Autodesk Inventor part; units mm, degrees
(part 4 of 4)
  arc A561 (-1.6111, 29.8706) -> (-1.4437, 30.2273) centre (-7.325, 32.7708) ccw
  arc A562 (-1.4437, 30.2273) -> (-1.2651, 30.6794) centre (-8.4075, 33.2394) ccw
  arc A563 (-1.2651, 30.6794) -> (-1.5585, 30.9505) centre (-15.3265, 15.7621) ccw
  arc A564 (-1.5585, 30.9505) -> (-1.9952, 30.737) centre (1.554, 24.031) ccw
  arc A565 (-1.9952, 30.737) -> (-2.3376, 30.5421) centre (1.0019, 25.0734) ccw
  arc A566 (-2.3376, 30.5421) -> (-2.5999, 30.3711) centre (0.4096, 26.0425) ccw
  arc A567 (-2.5999, 30.3711) -> (-2.8883, 30.6174) centre (-15.3265, 15.7621) ccw
  arc A568 (-2.8883, 30.6174) -> (-2.7604, 30.9032) centre (-7.6343, 32.9126) ccw
  arc A569 (-2.7604, 30.9032) -> (-2.6214, 31.2719) centre (-8.6842, 33.3461) ccw
  arc A570 (-2.6214, 31.2719) -> (-2.4789, 31.7366) centre (-9.8001, 33.7284) ccw
  arc A571 (-2.4789, 31.7366) -> (-2.7926, 31.984) centre (-15.3265, 15.7621) ccw
  arc A572 (-2.7926, 31.984) -> (-3.2112, 31.7368) centre (0.8532, 25.33) ccw
  arc A573 (-3.2112, 31.7368) -> (-3.5372, 31.5157) centre (0.221, 26.3258) ccw
  arc A574 (-3.5372, 31.5157) -> (-3.7853, 31.3246) centre (-0.4455, 27.2455) ccw
  arc A575 (-3.7853, 31.3246) -> (-4.0922, 31.5475) centre (-15.3265, 15.7621) ccw
  arc A576 (-4.0922, 31.5475) -> (-3.9871, 31.8425) centre (-9.0037, 33.4633) ccw
  arc A577 (-3.9871, 31.8425) -> (-3.8775, 32.2209) centre (-10.0843, 33.8131) ccw
  arc A578 (-3.8775, 32.2209) -> (-3.7718, 32.6954) centre (-11.2268, 34.1066) ccw
  arc A579 (-3.7718, 32.6954) -> (-4.104, 32.9173) centre (-15.3265, 15.7621) ccw
  arc A580 (-4.104, 32.9173) -> (-4.5019, 32.6381) centre (0.0527, 26.5699) ccw
  arc A581 (-4.5019, 32.6381) -> (-4.8096, 32.3921) centre (-0.6557, 27.5131) ccw
  arc A582 (-4.8096, 32.3921) -> (-5.0419, 32.1821) centre (-1.3924, 28.3776) ccw
  arc A583 (-5.0419, 32.1821) -> (-5.3653, 32.3803) centre (-15.3265, 15.7621) ccw
  arc A584 (-5.3653, 32.3803) -> (-5.2837, 32.6826) centre (-10.412, 33.9048) ccw
  arc A585 (-5.2837, 32.6826) -> (-5.2041, 33.0685) centre (-11.5167, 34.1687) ccw
  arc A586 (-5.2041, 33.0685) -> (-5.136, 33.5498) centre (-12.6787, 34.3717) ccw
  arc A587 (-5.136, 33.5498) -> (-5.4845, 33.745) centre (-15.3265, 15.7621) ccw
  arc A588 (-5.4845, 33.745) -> (-5.8594, 33.4354) centre (-0.8427, 27.7432) ccw
  arc A589 (-5.8594, 33.4354) -> (-6.1468, 33.166) centre (-1.6229, 28.628) ccw
  arc A590 (-6.1468, 33.166) -> (-6.3619, 32.9384) centre (-2.4252, 29.432) ccw
  arc A591 (-6.3619, 32.9384) -> (-6.6999, 33.1106) centre (-15.3265, 15.7621) ccw
  arc A592 (-6.6999, 33.1106) -> (-6.6422, 33.4184) centre (-11.8506, 34.2345) ccw
  arc A593 (-6.6422, 33.4184) -> (-6.5932, 33.8093) centre (-12.9726, 34.4109) ccw
  arc A594 (-6.5932, 33.8093) -> (-6.563, 34.2945) centre (-14.147, 34.5221) ccw
  arc A595 (-6.563, 34.2945) -> (-6.9258, 34.4617) centre (-15.3265, 15.7621) ccw
  arc A596 (-6.9258, 34.4617) -> (-7.2752, 34.1237) centre (-1.8274, 28.8427) ccw
  arc A597 (-7.2752, 34.1237) -> (-7.5406, 33.8326) centre (-2.6746, 29.6635) ccw
  arc A598 (-7.5406, 33.8326) -> (-7.7372, 33.5888) centre (-3.5375, 30.4021) ccw
  arc A599 (-7.7372, 33.5888) -> (-8.0876, 33.7339) centre (-15.3265, 15.7621) ccw
  arc A600 (-8.0876, 33.7339) -> (-8.0543, 34.0453) centre (-13.3106, 34.4503) ccw
  arc A601 (-8.0543, 34.0453) -> (-8.0361, 34.4389) centre (-14.443, 34.5381) ccw
  arc A602 (-8.0361, 34.4389) -> (-8.0441, 34.9249) centre (-15.6225, 34.5568) ccw
  arc A603 (-8.0441, 34.9249) -> (-8.4189, 35.0632) centre (-15.3265, 15.7621) ccw
  arc A604 (-8.4189, 35.0632) -> (-8.7406, 34.6988) centre (-2.8953, 29.8615) ccw
  arc A605 (-8.7406, 34.6988) -> (-8.9824, 34.3877) centre (-3.8043, 30.6133) ccw
  arc A606 (-8.9824, 34.3877) -> (-9.1593, 34.1293) centre (-4.7224, 31.2819) ccw
  arc A607 (-9.1593, 34.1293) -> (-9.52, 34.2465) centre (-15.3265, 15.7621) ccw
  arc A608 (-9.52, 34.2465) -> (-9.5112, 34.5595) centre (-14.7831, 34.5508) ccw
  arc A609 (-9.5112, 34.5595) -> (-9.5239, 34.9533) centre (-15.9189, 34.5495) ccw
  arc A610 (-9.5239, 34.9533) -> (-9.57, 35.4372) centre (-17.0962, 34.4756) ccw
  arc A611 (-9.57, 35.4372) -> (-9.9545, 35.5457) centre (-15.3265, 15.7621) ccw
  arc A612 (-9.9545, 35.5457) -> (-10.2467, 35.1572) centre (-4.0399, 30.7934) ccw
  arc A613 (-10.2467, 35.1572) -> (-10.4633, 34.8281) centre (-5.005, 31.4715) ccw
  arc A614 (-10.4633, 34.8281) -> (-10.6194, 34.5566) centre (-5.9728, 32.0661) ccw
  arc A615 (-10.6194, 34.5566) -> (-10.9881, 34.6451) centre (-15.3265, 15.7621) ccw
  arc A616 (-10.9881, 34.6451) -> (-11.0039, 34.9579) centre (-16.2589, 34.5355) ccw
  arc A617 (-11.0039, 34.9579) -> (-11.0475, 35.3494) centre (-17.3911, 34.4452) ccw
  arc A618 (-11.0475, 35.3494) -> (-11.1315, 35.8282) centre (-18.559, 34.2791) ccw
  arc A619 (-11.1315, 35.8282) -> (-11.5233, 35.9062) centre (-15.3265, 15.7621) ccw
  arc A620 (-11.5233, 35.9062) -> (-11.7841, 35.4959) centre (-5.254, 31.6326) ccw
  arc A621 (-11.7841, 35.4959) -> (-11.9742, 35.1509) centre (-6.2694, 32.2329) ccw
  arc A622 (-11.9742, 35.1509) -> (-12.1085, 34.8679) centre (-7.2808, 32.7497) ccw
  arc A623 (-12.1085, 34.8679) -> (-12.4831, 34.9273) centre (-15.3265, 15.7621) ccw
  arc A624 (-12.4831, 34.9273) -> (-12.5234, 35.2378) centre (-17.729, 34.4045) ccw
  arc A625 (-12.5234, 35.2378) -> (-12.5975, 35.6248) centre (-18.8506, 34.2256) ccw
  arc A626 (-12.5975, 35.6248) -> (-12.7188, 36.0955) centre (-20.0019, 33.9684) ccw
  arc A627 (-12.7188, 36.0955) -> (-13.1155, 36.1425) centre (-15.3265, 15.7621) ccw
  arc A628 (-13.1155, 36.1425) -> (-13.3433, 35.713) centre (-6.5302, 32.3739) ccw
  arc A629 (-13.3433, 35.713) -> (-13.5057, 35.3541) centre (-7.5896, 32.8927) ccw
  arc A630 (-13.5057, 35.3541) -> (-13.6174, 35.0615) centre (-8.6385, 33.3286) ccw
  arc A631 (-13.6174, 35.0615) -> (-13.9955, 35.0913) centre (-15.3265, 15.7621) ccw
  arc A632 (-13.9955, 35.0913) -> (-14.0601, 35.3977) centre (-19.1843, 34.1586) ccw
  arc A633 (-14.0601, 35.3977) -> (-14.1644, 35.7777) centre (-20.2884, 33.8922) ccw
  arc A634 (-14.1644, 35.7777) -> (-14.3222, 36.2374) centre (-21.4159, 33.5455) ccw
  arc A635 (-14.3222, 36.2374) -> (-14.7213, 36.2531) centre (-15.3265, 15.7621) ccw
  arc A636 (-14.7213, 36.2531) -> (-14.9147, 35.8071) centre (-7.8607, 33.0129) ccw
  arc A637 (-14.9147, 35.8071) -> (-15.0485, 35.4366) centre (-8.9575, 33.447) ccw
  arc A638 (-15.0485, 35.4366) -> (-15.1369, 35.1361) centre (-10.0373, 33.7992) ccw
  arc A639 (-15.1369, 35.1361) -> (-15.5162, 35.1361) centre (-15.3265, 15.7621) ccw
  circle A640 centre (-15.3265, 15.7621) radius 18.25
  point P0 (0, 0)
  dimension "d5" = 36.5
  constraints: 1 centre point, 1 coincident
  measures "d5" diameter of A640
extrude "押し出し3" cut sketch "スケッチ3" against normal blind 0.75 contours A640
sketch "スケッチ4" plane through (15.3265, 15.7621, 2.25) normal (0, 0, 1) x (1, 0, 0)
  circle A0 centre (0, 0) radius 18.25
  circle A1 centre (0, 0) radius 17
  line L0 (0, 14) -> (12.1244, -7) construction
  line L1 (12.1244, -7) -> (-12.1244, -7) construction
  line L2 (-12.1244, -7) -> (0, 14) construction
  circle A2 centre (0, 14) radius 1.5
  circle A3 centre (-12.1244, -7) radius 1.5
  circle A4 centre (12.1244, -7) radius 1.5
  circle A5 centre (0, 14) radius 3
  circle A6 centre (-12.1244, -7) radius 3
  circle A7 centre (12.1244, -7) radius 3
  point P0 (-15.3265, -15.7621)
  dimension "d8" = 34
  dimension "d9" = 3
  dimension "d10" = 3
  dimension "d11" = 3
  dimension "d12" = 6
  dimension "d13" = 6
  dimension "d14" = 6
  dimension "d30" = 14
  constraints: 8 coincident, 7 centre point, 6 end point, 1 horizontal, 1 tangent, 7 other
  measures "d8" diameter of A1
  measures "d9" diameter of A2
  measures "d10" diameter of A3
  measures "d11" diameter of A4
  measures "d12" diameter of A5
  measures "d13" diameter of A6
  measures "d14" diameter of A7
  measures "d30" distance of A0.centre L0.start
extrude "押し出し4" cut sketch "スケッチ4" against normal through all contours A2 | A3 | A4
sketch "スケッチ5" plane through (15.3265, 15.7621, 0.75) normal (0, 0, -1) x (-1, 0, 0)
  circle A0 centre (12.1244, -7) radius 1.5
  circle A1 centre (0, 14) radius 1.5
  circle A2 centre (-12.1244, -7) radius 1.5
  circle A3 centre (0, 0) radius 18.25
  arc A4 (-9.2773, -10.4848) -> (9.2773, -10.4848) centre (0, 0) ccw
  arc A5 (13.7188, -2.7919) -> (4.4415, 13.2768) centre (0, 0) ccw
  arc A6 (-4.4415, 13.2768) -> (-13.7188, -2.7919) centre (0, 0) ccw
  arc A7 (1.6868, 18.1719) -> (-1.6868, 18.1719) centre (0, 14) ccw
  arc A8 (-4.4415, 13.2768) -> (4.4415, 13.2768) centre (0, 14) ccw
  arc A9 (13.7188, -2.7919) -> (9.2773, -10.4848) centre (12.1244, -7) ccw
  arc A10 (14.8939, -10.5468) -> (16.5807, -7.6251) centre (12.1244, -7) ccw
  arc A11 (-9.2773, -10.4848) -> (-13.7188, -2.7919) centre (-12.1244, -7) ccw
  arc A12 (-16.5807, -7.6251) -> (-14.8939, -10.5468) centre (-12.1244, -7) ccw
  point P0 (15.3265, -15.7621)
  dimension "d21" = 14
  dimension "d22" = 14
  dimension "d23" = 14
  dimension "d24" = 3
  dimension "d25" = 3
  dimension "d26" = 3
  constraints: 24 point on circle, 9 centre point, 1 coincident
  measures "d21" radius of A4
  measures "d22" radius of A6
  measures "d23" radius of A5
  measures "d24" radial gap between concentric circles of A0 A9
  measures "d25" radial gap between concentric circles of A2 A11
  measures "d26" radial gap between concentric circles of A8 A1
extrude "押し出し5" cut sketch "スケッチ5" against normal through all contours A11 A6 A8 A5 A9 A4
fillet "フィレット1" radius 1 6 edges at (1.6078, 12.9701, 1.5) (6.0493, 5.2772, 1.5) (24.6038, 5.2772, 1.5) (29.0453, 12.9701, 1.5) (19.768, 29.0389, 1.5) (10.885, 29.0389, 1.5)
